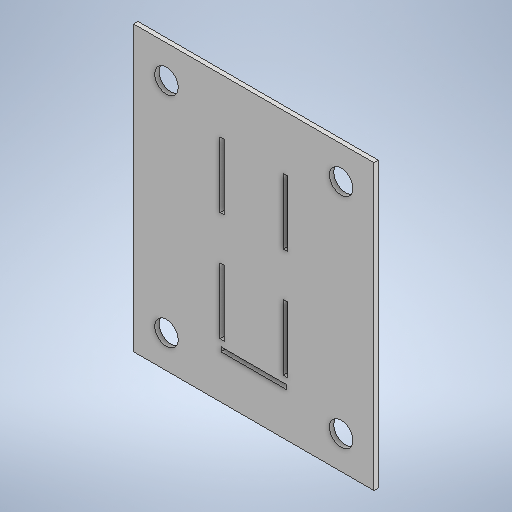
# Autodesk Inventor part: Piston_FloorHinge_BasePlate
Saved by Autodesk Inventor 2025.2 (Build 292293000, 293)
## iProperties
Created: 2025-04-08
Part Number: Piston_FloorHinge_BasePlate
Material: Generic
Document SubType Name: Sheet Metal
Designer: Victor
Density: 1 g/cm^3
Sheet Metal Rule: Default_mm
Appearance: Default
Author: Victor
Autodesk Inventor part; units mm, degrees
ref_plane "YZ Plane" through (0, 0, 0) normal (1, 0, 0) x (0, 1, 0)
ref_plane "XZ Plane" through (0, 0, 0) normal (0, 1, 0) x (-1, 0, 0)
ref_plane "XY Plane" through (0, 0, 0) normal (0, 0, 1) x (1, 0, 0)
sketch "Sketch1" plane through (0, 0, 0) normal (0, 0, 1) x (1, 0, 0)
  line L0 (-55, 0) -> (55, 0)
  line L1 (55, 0) -> (55, -130)
  line L2 (55, -130) -> (-55, -130)
  line L3 (-55, -130) -> (-55, 0)
  line L4 (0, 0) -> (0, -130)
  line L5 (-55, -65) -> (55, -65)
  circle A0 centre (40, -15) radius 5.35
  line L6 (55, -65) -> (-55, -65)
  circle A1 centre (-40, -15) radius 5.35
  circle A2 centre (40, -115) radius 5.35
  circle A3 centre (-40, -115) radius 5.35
  dimension "d0" = 110
  dimension "d1" = 130
  dimension "d2" = 10.7
  dimension "d3" = 40
  dimension "d4" = 50
  measures "d0" distance of L1.end L2.end
  measures "d1" distance of L0.end L1.end
  measures "d2" diameter of A0
  measures "d3" distance from line of L4 A0.centre
  measures "d4" distance from line of L5 A0.centre
extrude "Plate1" add sketch "Sketch1" along normal blind 2
sketch "Sketch2" plane through (0, 0, 2) normal (0, 0, 1) x (1, 0, 0)
  line L0 (13.5, -25) -> (15.5, -25)
  line L1 (15.5, -25) -> (15.5, -55)
  line L2 (15.5, -55) -> (13.5, -55)
  line L3 (13.5, -55) -> (13.5, -25)
  line L4 (0, 0) -> (0, -130)
  line L5 (-55, -130) -> (55, -130) projected
  line L6 (-55, 0) -> (55, 0) projected
  line L7 (-55, 0) -> (-55, -130) projected
  line L8 (-55, -65) -> (55, -65)
  line L9 (55, -130) -> (55, 0) projected
  line L10 (13.5, -105) -> (15.5, -105)
  line L11 (15.5, -105) -> (15.5, -75)
  line L12 (15.5, -75) -> (13.5, -75)
  line L13 (13.5, -75) -> (13.5, -105)
  line L14 (-13.5, -25) -> (-15.5, -25)
  line L15 (-15.5, -25) -> (-15.5, -55)
  line L16 (-15.5, -55) -> (-13.5, -55)
  line L17 (-13.5, -55) -> (-13.5, -25)
  line L18 (-13.5, -75) -> (-13.5, -105)
  line L19 (-15.5, -105) -> (-15.5, -75)
  line L20 (-13.5, -105) -> (-15.5, -105)
  line L21 (-15.5, -75) -> (-13.5, -75)
  line L22 (-15, -108) -> (15, -108)
  line L23 (15, -108) -> (15, -110)
  line L24 (15, -110) -> (-15, -110)
  line L25 (-15, -110) -> (-15, -108)
  point P0 (13.5, -40)
  point P1 (14.5, -25)
  point P2 (-15, -109)
  dimension "d6" = 2
  dimension "d7" = 30
  dimension "d8" = 13.5
  dimension "d9" = 25
  dimension "d10" = 30
  dimension "d11" = 2
  dimension "d12" = 15
  dimension "d13" = 20
  constraints: 44 end point, 12 symmetric about line, 6 midpoint, 4 parallel, 2 horizontal, 2 perpendicular
  measures "d6" distance of L1.end L2.end
  measures "d7" distance of L0.end L1.end
  measures "d8" distance from line of point (13.5, -40) L4
  measures "d9" distance from line of L6 point (14.5, -25)
  measures "d10" distance of L23.end L24.end
  measures "d11" distance of L22.end L23.end
  measures "d12" distance from line of L4 point (-15, -109)
  measures "d13" distance between parallel lines of L5 L24
extrude "Cut1" cut sketch "Sketch2" against normal blind 2 contours L0 L1 L2 L3 | L22 L23 L24 L4 | L4 L24 L25 L22 | L13 L12 L11 L10 | L17 L16 L15 L14 | L18 L20 L19 L21
equation "\"d6\" = plate_thickness"
equation "\"d8\" = 0.5 * L_Piston_Bottom + A_joint_tolerance"
equation "\"d11\" = plate_thickness"
equation "\"d14\" = Thickness"
equation "\"d5\" = Thickness"
equation "\"Thickness\" = plate_thickness"
equation "\"BendRadius\" = Thickness"
equation "\"BendReliefWidth\" = Thickness"
equation "\"BendReliefDepth\" = 0.5 * Thickness"
equation "\"CornerReliefSize\" = 4 * Thickness"
equation "\"MinimumRemnant\" = 2 * Thickness"
equation "\"TransitionRadius\" = BendRadius"
equation "\"JacobiRadiusSize\" = BendRadius"
equation "\"GapSize\" = Thickness"
equation "\"A_joint_tolerance\" = 3"
equation "\"l___________\" = 0"
equation "\"l__________\" = 0"
equation "\"l_________\" = 0"
equation "\"rivet_diameter\" = 4"
equation "\"plate_thickness\" = 2"
equation "\"l________\" = 0"
equation "\"L_Piston_Bottom\" = 21"
equation "\"L_Piston_Top\" = 25"
body "Solid1"
